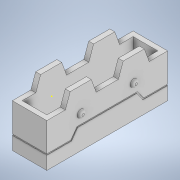
# Autodesk Inventor part: blade connector
Saved by Autodesk Inventor 2021 (Build 250183000, 183)
## iProperties
Created: 2021-03-29
Part Number: blade connector
Material: Generic
Document SubType Name: Modeling
Designer: newic
Density: 1 g/cm^3
Appearance: Default
Author: newic
Autodesk Inventor part; units mm, degrees
ref_plane "YZ Plane" through (0, 0, 0) normal (1, 0, 0) x (0, 1, 0)
ref_plane "XZ Plane" through (0, 0, 0) normal (0, 1, 0) x (-1, 0, 0)
ref_plane "XY Plane" through (0, 0, 0) normal (0, 0, 1) x (1, 0, 0)
sketch "Sketch1" plane through (0, 0, 0) normal (0, 1, 0) x (-1, 0, 0)
  line L0 (0, 0) -> (12.7, 0)
  line L1 (12.7, 0) -> (12.7, -57.15)
  line L2 (12.7, -57.15) -> (0, -57.15)
  line L3 (0, -57.15) -> (0, 0)
  line L4 (15.24, -59.69) -> (15.24, 2.54)
  line L5 (15.24, 2.54) -> (-2.54, 2.54)
  line L6 (-2.54, 2.54) -> (-2.54, -59.69)
  line L7 (-2.54, -59.69) -> (15.24, -59.69)
  dimension "d0" = 12.7
  dimension "d1" = 57.15
  dimension "d2" = 2.54
  constraints: 16 end point, 4 parallel, 2 perpendicular, 1 horizontal, 3 other
  measures "d0" distance of L1.end L2.end
  measures "d1" distance of L0.end L1.end
  measures "d2" distance between parallel lines of L1 L4
extrude "Extrusion1" add sketch "Sketch1" against normal blind 31.75
sketch "Sketch2" plane through (2.54, 0, 2.54) normal (1, 0, 0) x (0, 0, -1)
  point P0 (2.54, 0)
sketch "Sketch3" plane through (2.54, 0, 2.54) normal (1, 0, 0) x (0, 0, -1)
  line L0 (59.69, 0) -> (2.54, 0) projected
  line L1 (-1.2014, -9.525) -> (66.2927, -9.525)
  line L2 (31.115, 0) -> (31.115, -9.525)
  line L3 (0, 0) -> (0, -31.75) projected
  line L4 (0, -9.525) -> (8.255, -9.525)
  line L5 (62.23, 0) -> (62.23, -31.75) projected
  line L6 (62.23, -9.525) -> (53.975, -9.525)
  line L7 (31.115, -9.525) -> (34.925, -9.525)
  line L8 (31.115, -9.525) -> (27.305, -9.525)
  line L9 (0, -9.525) -> (9.525, -9.525)
  line L10 (31.115, -9.525) -> (25.4, -9.525)
  line L11 (31.115, -9.525) -> (36.83, -9.525)
  line L12 (62.23, -9.525) -> (52.705, -9.525)
  line L13 (0, 5.2281) -> (17.78, 5.2281)
  line L14 (17.78, 5.2281) -> (17.78, -9.525)
  line L15 (17.78, 0) -> (17.78, -2.54)
  line L16 (0, -2.54) -> (62.23, -2.54)
  line L17 (36.83, -9.525) -> (44.4179, 11.3227)
  line L18 (52.705, -9.525) -> (48.1245, 3.0598)
  line L19 (9.525, -9.525) -> (14.5428, 4.2614)
  line L20 (25.4, -9.525) -> (21.085, 2.3303)
  line L21 (36.83, -9.525) -> (52.705, -9.525)
  line L22 (-3.8276, -2.6318) -> (67.8028, -2.6318)
  line L23 (67.8028, -2.6318) -> (67.8028, 7.3948)
  line L24 (67.8028, 7.3948) -> (-3.8276, 7.3948)
  line L25 (-3.8276, 7.3948) -> (-3.8276, -2.6318)
  line L26 (-1.2014, -9.525) -> (-3.8276, -2.6318)
  line L27 (65.275, -9.525) -> (67.8028, -2.6318)
  point P0 (12.0339, -2.6318)
  point P1 (22.8911, -2.6318)
  point P2 (39.3389, -2.6318)
  point P3 (50.1961, -2.6318)
  dimension "d10" = 9.525
  dimension "d11" = 5.715
  dimension "d12" = 5.715
  dimension "d13" = 9.525
  dimension "d14" = 17.78
  dimension "d15" = 2.54
  dimension "d16" = 70
  dimension "d17" = 70
  dimension "d18" = 70
  dimension "d19" = 70
  constraints: 48 end point, 8 point on line, 3 horizontal, 2 parallel, 2 perpendicular, 2 vertical, 1 midpoint, 16 other
  measures "d10" distance of L4.start L9.end
  measures "d11" distance of L2.end L10.end
  measures "d12" distance of L2.end L11.end
  measures "d13" distance of L6.start L12.end
  measures "d14" distance of L13.start L13.end
  measures "d15" distance of L15.start L15.end
  measures "d16" angle to the sketch x axis of L19
  measures "d17" angle to the sketch x axis of L20
  measures "d18" angle to the sketch x axis of L17
  measures "d19" angle to the sketch x axis of L18
extrude "Extrusion2" cut sketch "Sketch3" against normal through all contours L18 L16 L17 L0 | L0 L17 L24 L23 L22 L5 L16 L18 | L17 L16 L2 L0 | L0 L19 L16 L3 L22 L25 L24 L17 | L18 L22 L17 L16 | L16 L5 L22 L18 | L2 L16 L20 L0 | L17 L22 L2 L16 | L22 L5 L1 L18 | L20 L16 L14 L0 | L2 L22 L20 L16 | L17 L1 L2 L22 | L22 L27 L1 L5 | L14 L16 L19 L0 | L20 L22 L14 L16 | L2 L1 L20 L22 | L22 L3 L1 L26 | L14 L22 L19 L16 | L22 L19 L1 L3 | L3 L16 L19 L22
sketch "Sketch4" plane through (2.54, -31.75, 2.54) normal (1, 0, 0) x (0, 0, -1)
  line L0 (0, 22.225) -> (0, 0) projected
  line L1 (0, 22.225) -> (0, 0)
  line L2 (0, 0) -> (0, 7.366)
  line L3 (0, 7.366) -> (62.23, 7.366)
  line L4 (62.23, 22.225) -> (62.23, 0) projected
  line L5 (12.0339, 29.1182) -> (22.8911, 29.1182) projected
  line L6 (17.4625, 29.1182) -> (17.4625, 4.5442)
  line L7 (50.1961, 29.1182) -> (39.3389, 29.1182) projected
  line L8 (44.7675, 29.1182) -> (44.7675, 5.1393)
  line L9 (17.4625, 7.366) -> (14.2875, 7.366)
  line L10 (44.7675, 7.366) -> (47.9425, 7.366)
  line L11 (47.9425, 7.366) -> (47.9425, 11.811)
  line L12 (14.2875, 7.366) -> (14.2875, 11.811)
  line L13 (17.4625, 11.811) -> (44.7675, 11.811)
  line L14 (0, 7.366) -> (0, 22.225)
  line L15 (0, 14.7955) -> (64.3687, 14.7955)
  line L16 (0, 16.7005) -> (64.3687, 16.7005)
  circle A0 centre (17.4625, 16.7005) radius 1.905
  circle A1 centre (44.7675, 16.7005) radius 1.905
  line L17 (46.6725, 11.811) -> (49.8475, 7.366)
  line L18 (15.5575, 11.811) -> (12.3825, 7.366)
  line L19 (15.5575, 11.811) -> (17.4625, 11.811)
  line L20 (46.6725, 11.811) -> (44.7675, 11.811)
  line L21 (12.8992, 6.9969) -> (15.8843, 11.176)
  line L22 (15.8843, 11.176) -> (17.4625, 11.176)
  line L23 (17.4625, 11.176) -> (44.7675, 11.176)
  line L24 (44.7675, 11.176) -> (46.3457, 11.176)
  line L25 (46.3457, 11.176) -> (49.3308, 6.9969)
  line L26 (0, 6.731) -> (62.23, 6.731)
  line L27 (12.8992, 6.9969) -> (12.7093, 6.731)
  line L28 (49.3308, 6.9969) -> (49.8475, 6.3495)
  point P0 (2.54, 31.75)
  point P1 (49.543, 6.731)
  point P2 (62.23, 6.731)
  point P3 (0, 7.366)
  point P4 (0, 6.731)
  dimension "d22" = 7.366
  dimension "d23" = 3.175
  dimension "d24" = 3.175
  dimension "d25" = 4.445
  dimension "d26" = 4.445
  dimension "d27" = 1.905
  dimension "d28" = 0.635
  dimension "d29" = 0.635
  constraints: 50 end point, 17 point on line, 4 perpendicular, 3 midpoint, 3 vertical, 2 centre point, 2 collinear, 2 parallel, 4 other
  measures "d22" distance of L0.end L2.end
  measures "d23" distance of L9.start L9.end
  measures "d24" distance of L10.start L10.end
  measures "d25" distance of L10.end L11.end
  measures "d26" distance of L9.end L12.end
  measures "d27" distance between parallel lines of L15 L16
  measures "d28" distance between parallel lines of L18 L21
  measures "d29" distance between parallel lines of L3 L26
sketch "Sketch5" plane through (-15.24, -31.75, -59.69) normal (-1, 0, 0) x (0, 0, 1)
  line L0 (0, 22.225) -> (0, 0)
  line L1 (0, 22.225) -> (0, 0)
  line L2 (0, 0) -> (0, 7.366)
  line L3 (0, 7.366) -> (62.23, 7.366)
  line L4 (62.23, 22.225) -> (62.23, 0)
  line L5 (12.0339, 29.1182) -> (22.8911, 29.1182)
  line L6 (17.4625, 29.1182) -> (17.4625, 4.5442)
  line L7 (50.1961, 29.1182) -> (39.3389, 29.1182)
  line L8 (44.7675, 29.1182) -> (44.7675, 5.1393)
  line L9 (17.4625, 7.366) -> (14.2875, 7.366)
  line L10 (44.7675, 7.366) -> (47.9425, 7.366)
  line L11 (47.9425, 7.366) -> (47.9425, 11.811)
  line L12 (14.2875, 7.366) -> (14.2875, 11.811)
  line L13 (17.4625, 11.811) -> (44.7675, 11.811)
  line L14 (0, 7.366) -> (0, 22.225)
  line L15 (0, 14.7955) -> (64.3687, 14.7955)
  line L16 (0, 16.7005) -> (64.3687, 16.7005)
  circle A0 centre (17.4625, 16.7005) radius 1.905
  circle A1 centre (44.7675, 16.7005) radius 1.905
  line L17 (46.6725, 11.811) -> (49.8475, 7.366)
  line L18 (15.5575, 11.811) -> (12.3825, 7.366)
  line L19 (15.5575, 11.811) -> (17.4625, 11.811)
  line L20 (46.6725, 11.811) -> (44.7675, 11.811)
  line L21 (12.8992, 6.9969) -> (15.8843, 11.176)
  line L22 (15.8843, 11.176) -> (17.4625, 11.176)
  line L23 (17.4625, 11.176) -> (44.7675, 11.176)
  line L24 (44.7675, 11.176) -> (46.3457, 11.176)
  line L25 (46.3457, 11.176) -> (49.3308, 6.9969)
  line L26 (0, 6.731) -> (62.23, 6.731)
  line L27 (12.8992, 6.9969) -> (12.7093, 6.731)
  line L28 (49.3308, 6.9969) -> (49.8475, 6.3495)
  point P0 (59.69, 31.75)
  point P1 (2.54, 31.75)
  point P2 (0, 6.731)
  point P3 (49.543, 6.731)
  point P4 (62.23, 6.731)
  point P5 (0, 7.366)
  dimension "d30" = 7.366
  dimension "d31" = 3.175
  dimension "d32" = 3.175
  dimension "d33" = 4.445
  dimension "d34" = 4.445
  dimension "d35" = 1.905
  dimension "d36" = 0.635
  dimension "d37" = 0.635
  constraints: 58 end point, 17 point on line, 4 perpendicular, 3 midpoint, 3 vertical, 2 centre point, 2 collinear, 2 parallel, 4 other
  measures "d30" distance of L0.end L14.start
  measures "d31" distance of L9.start L9.end
  measures "d32" distance of L10.start L10.end
  measures "d33" distance of L10.end L11.end
  measures "d34" distance of L9.end L12.end
  measures "d35" distance between parallel lines of L15 L16
  measures "d36" distance between parallel lines of L18 L21
  measures "d37" distance between parallel lines of L3 L26
extrude "Extrusion3" cut sketch "Sketch5" against normal blind 0.254 contours L3 L21 L27 L26 L0 | L18 L12 L21 L3 | L13 L8 L23 L6 | L6 L22 L21 L12 L18 L19 | L20 L17 L11 L25 L24 L8 | L4 L26 L28 L25 L3 | L17 L3 L25 L11
sketch "Sketch6" plane through (-15.24, -9.525, -34.29) normal (-1, 0, 0) x (0, 0, 1)
  line L0 (-25.4, 0) -> (-25.4, -22.225)
  line L1 (-25.4, 0) -> (-25.4, -22.225)
  line L2 (-25.4, -22.225) -> (-25.4, -14.859)
  line L3 (-25.4, -14.859) -> (36.83, -14.859)
  line L4 (36.83, 0) -> (36.83, -22.225)
  line L5 (-13.3661, 6.8933) -> (-2.5089, 6.8933)
  line L6 (-7.9375, 6.8933) -> (-7.9375, -17.6808)
  line L7 (24.7961, 6.8933) -> (13.9389, 6.8933)
  line L8 (19.3675, 6.8933) -> (19.3675, -17.0857)
  line L9 (-7.9375, -14.859) -> (-11.1125, -14.859)
  line L10 (19.3675, -14.859) -> (22.5425, -14.859)
  line L11 (22.5425, -14.859) -> (22.5425, -10.414)
  line L12 (-11.1125, -14.859) -> (-11.1125, -10.414)
  line L13 (-7.9375, -10.414) -> (19.3675, -10.414)
  line L14 (-25.4, -14.859) -> (-25.4, 0)
  line L15 (-25.4, -7.4295) -> (38.9686, -7.4295)
  line L16 (-25.4, -5.5245) -> (38.9686, -5.5245)
  circle A0 centre (-7.9375, -5.5245) radius 1.905
  circle A1 centre (19.3675, -5.5245) radius 1.905
  line L17 (21.2725, -10.414) -> (24.4475, -14.859)
  line L18 (-9.8425, -10.414) -> (-13.0175, -14.859)
  line L19 (-9.8425, -10.414) -> (-7.9375, -10.414)
  line L20 (21.2725, -10.414) -> (19.3675, -10.414)
  line L21 (-12.5008, -15.228) -> (-9.5157, -11.049)
  line L22 (-9.5157, -11.049) -> (-7.9375, -11.049)
  line L23 (-7.9375, -11.049) -> (19.3675, -11.049)
  line L24 (19.3675, -11.049) -> (20.9457, -11.049)
  line L25 (20.9457, -11.049) -> (23.9308, -15.228)
  line L26 (-25.4, -15.494) -> (36.83, -15.494)
  line L27 (-12.5008, -15.228) -> (-12.6907, -15.494)
  line L28 (23.9308, -15.228) -> (24.4475, -15.8755)
  point P0 (34.29, 9.525)
  point P1 (-22.86, 9.525)
  dimension "d40" = 7.366
  dimension "d41" = 3.175
  dimension "d42" = 3.175
  dimension "d43" = 4.445
  dimension "d44" = 4.445
  dimension "d45" = 1.905
  dimension "d46" = 0.635
  dimension "d47" = 0.635
  constraints: 58 end point, 17 point on line, 4 perpendicular, 3 midpoint, 3 vertical, 2 centre point, 2 collinear, 2 parallel, 4 other
  measures "d40" distance of L0.end L3.start
  measures "d41" distance of L9.start L9.end
  measures "d42" distance of L10.start L10.end
  measures "d43" distance of L10.end L11.end
  measures "d44" distance of L9.end L12.end
  measures "d45" distance between parallel lines of L15 L16
  measures "d46" distance between parallel lines of L18 L21
  measures "d47" distance between parallel lines of L3 L26
extrude "Extrusion4" cut sketch "Sketch4" against normal blind 0.254 contours L3 L21 L27 L26 L0 | L18 L12 L21 L3 | L13 L8 L23 L6 | L6 L22 L21 L12 L18 L19 | L20 L17 L11 L25 L24 L8 | L4 L26 L28 L25 L3 | L17 L3 L25 L11
sketch "Sketch7" plane through (2.54, -9.525, -22.86) normal (1, 0, 0) x (0, 0, -1)
  point P0 (-22.86, 9.525)
extrude "Extrusion5" add sketch "Sketch6" along normal blind 1.27 contours A0 L6 L16 | L16 L6 A0 | L6 L16 A0 | L6 A0 L16 | A1 L16 L8 | L8 L16 A1 | L16 A1 L8 | L8 A1 L16
sketch "Sketch8" plane through (2.54, -9.525, -22.86) normal (1, 0, 0) x (0, 0, -1)
  circle A0 centre (-7.9375, -5.5245) radius 1.905 projected
  circle A1 centre (-7.9375, -5.5245) radius 1.905
  circle A2 centre (19.3675, -5.5245) radius 1.905 projected
  circle A3 centre (19.3675, -5.5245) radius 1.905
  point P0 (-22.86, 9.525)
  constraints: 2 centre point, 2 coincident
extrude "Extrusion6" add sketch "Sketch8" along normal blind 1.27
sketch "Sketch9" plane through (-15.24, -9.525, -34.29) normal (-1, 0, 0) x (0, 0, 1)
  line L0 (-25.4, 0) -> (-25.4, -14.859) projected
  line L1 (-25.4, -15.494) -> (-12.713, -15.494) projected
  line L2 (-25.4, -14.859) -> (-25.146, -14.859)
  line L3 (-25.146, -14.859) -> (-25.146, -15.494)
  line L4 (-25.146, -15.494) -> (-25.4, -15.494)
  line L5 (-25.4, -15.494) -> (-25.4, -14.859)
  line L6 (24.4475, -14.859) -> (36.83, -14.859) projected
  line L7 (36.83, -15.494) -> (36.576, -15.494)
  line L8 (36.576, -15.494) -> (36.576, -14.859)
  line L9 (36.576, -14.859) -> (36.83, -14.859)
  line L10 (36.83, -14.859) -> (36.83, -15.494)
  point P0 (34.29, 9.525)
  dimension "d54" = 0.254
  dimension "d55" = 0.254
  constraints: 16 end point, 4 parallel, 2 horizontal, 2 perpendicular, 2 point on line
  measures "d54" distance of L3.end L4.end
  measures "d55" distance of L8.end L9.end
extrude "Extrusion7" cut sketch "Sketch9" against normal blind 2540
fillet "Fillet1" radius 1.27 4 edges at (-16.51, -15.0495, -44.1325) (-16.51, -15.0495, -16.8275) (3.81, -15.0495, -13.0175) (3.81, -15.0495, -40.3225)
body "Solid1"
